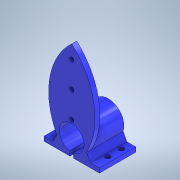
# Autodesk Inventor part: Soporte_MotorDC
Saved by Autodesk Inventor 2022 (Build 260153000, 153)
## iProperties
Created: 2022-01-28
Part Number: Soporte_MotorDC
Material: ABS Plastic
Document SubType Name: Modeling
Designer: hurta
Density: 1.06 g/cm^3
Appearance: Blue - Wall Paint - Glossy
Author: hurta
Autodesk Inventor part; units mm, degrees
ref_plane "YZ Plane" through (0, 0, 0) normal (1, 0, 0) x (0, 1, 0)
ref_plane "XZ Plane" through (0, 0, 0) normal (0, 1, 0) x (-1, 0, 0)
ref_plane "XY Plane" through (0, 0, 0) normal (0, 0, 1) x (1, 0, 0)
sketch "Sketch1" plane through (0, 0, 0) normal (0, 0, 1) x (1, 0, 0)
  line L0 (10.7443, -13.75) -> (30.7443, -13.75)
  line L1 (30.7443, -13.75) -> (30.7443, -18.75)
  line L2 (-30.7443, -13.75) -> (-10.7443, -13.75)
  circle A0 centre (0, 0) radius 13.75
  arc A1 (10.7443, -13.75) -> (-10.7443, -13.75) centre (0, 0) ccw
  line L3 (-10.7443, -13.75) -> (10.7443, -13.75) construction
  line L4 (30.7443, -18.75) -> (-30.7443, -18.75)
  line L5 (-30.7443, -18.75) -> (-30.7443, -13.75)
  point P0 (-13.75, 0)
  dimension "d6" = 27.5
  dimension "d1" = 5
  dimension "d4" = 34.9
  dimension "d7" = 20
  constraints: 12 end point, 5 horizontal, 3 horizontal alignment, 2 coincident, 2 perpendicular, 2 point on circle, 1 centre point, 1 collinear, 2 other
  measures "d1" distance of L0.end L1.end
  measures "d4" diameter of A1
  measures "d7" distance of L2.start L2.end
extrude "Extrusion1" add sketch "Sketch1" along normal blind 35
sketch "Sketch2" plane through (-30.7443, -18.75, 0) normal (0, -1, 0) x (1, 0, 0)
  line L0 (0, 35) -> (61.4886, 35) projected
  line L1 (0, 0) -> (61.4886, 0) projected
  point P0 (30.7443, 0)
  point P1 (6.1489, 25)
  point P2 (55.3397, 25)
  point P3 (6.1489, 10)
  point P4 (55.3397, 10)
  dimension "d10" = 24.5954
  dimension "d11" = 61.4886
  dimension "d12" = 24.5954
  dimension "d13" = 10
  dimension "d14" = 10
  constraints: 2 horizontal alignment, 2 vertical alignment
  measures "d10" horizontal distance of point (6.149, 25) point (30.744, 0)
  measures "d11" distance of L0.start L0.end
  measures "d12" horizontal distance of point (30.744, 0) point (55.34, 25)
  measures "d13" distance from line of L0 point (6.149, 25)
  measures "d14" distance from line of L1 point (55.34, 10)
hole "Hole1" at (-24.5954, -18.75, 25) at (24.5954, -18.75, 25) at (-24.5954, -18.75, 10) at (24.5954, -18.75, 10) direction (0, 1, 0) diameter 5.5 end through all clearance for "Flat Head Machine Screw" size "M5" standard "Ansi Metric M Profile"
sketch "Sketch3" plane through (0, 0, 35) normal (0, 0, 1) x (1, 0, 0)
  line L0 (-2, -11.7546) -> (2, -11.7546)
  line L1 (2, -11.7546) -> (2, -18.75)
  line L2 (2, -18.75) -> (-2, -18.75)
  line L3 (-2, -18.75) -> (-2, -11.7546)
  line L4 (-30.7443, -18.75) -> (30.7443, -18.75) projected
  point P0 (0, 0)
  dimension "d22" = 2
  dimension "d23" = 2
  constraints: 8 end point, 2 parallel, 1 collinear, 1 horizontal, 1 perpendicular
  measures "d22" distance from line of point (0, 0) L1
  measures "d23" distance from line of point (0, 0) L3
extrude "Extrusion2" cut sketch "Sketch3" against normal through all
chamfer "Chamfer1" distance 10 angle 45 1 edges at (10.7443, -13.75, 17.5)
chamfer "Chamfer2" distance 10 angle 45 1 edges at (-10.7443, -13.75, 17.5)
sketch "Sketch4" plane through (0, 0, 35) normal (0, 0, 1) x (1, 0, 0)
  circle A0 centre (0, 17.45) radius 2.4
  circle A1 centre (0, 46.45) radius 2.4
  line L0 (2, -18.75) -> (30.7443, -18.75) projected
  arc A2 (16.5293, -5.5932) -> (-16.5293, -5.5932) centre (0, 0) ccw projected
  arc A3 (0, 90.45) -> (-16.5293, -5.5932) centre (54.2638, 31.6671) ccw
  arc A4 (16.5293, -5.5932) -> (0, 90.45) centre (-54.2638, 31.6671) ccw
  arc A5 (16.5293, -5.5932) -> (-16.5293, -5.5932) centre (0, 0) ccw projected
  arc A6 (2, -13.6038) -> (-2, -13.6038) centre (0, 0) ccw projected
  line L1 (-2, -18.75) -> (-2, -13.6038) projected
  line L2 (2, -13.6038) -> (2, -18.75) projected
  line L3 (30.7443, -18.75) -> (30.7443, -13.75) projected
  line L4 (30.7443, -13.75) -> (20.7443, -13.75) projected
  line L5 (16.5293, -5.5932) -> (20.7443, -13.75) projected
  line L6 (-20.7443, -13.75) -> (-16.5293, -5.5932) projected
  line L7 (-20.7443, -13.75) -> (-30.7443, -13.75) projected
  line L8 (-30.7443, -13.75) -> (-30.7443, -18.75) projected
  line L9 (-30.7443, -18.75) -> (-2, -18.75) projected
  circle A7 centre (0, 75.45) radius 2.4
  point P0 (16.5293, -5.5932)
  point P1 (-16.5293, -5.5932)
  dimension "d32" = 4.8
  dimension "d33" = 4.8
  dimension "d34" = 36.2
  dimension "d35" = 29
  dimension "d38" = 80
  dimension "d51" = 4.8
  dimension "d52" = 29
  dimension "d53" = 15
  dimension "d54" = 80
  constraints: 7 point on circle, 5 centre point, 4 vertical alignment, 3 coincident
  measures "d32" diameter of A0
  measures "d33" diameter of A1
  measures "d34" distance from line of L0 A0.centre
  measures "d35" distance of A1.centre A0.centre
  measures "d38" radius of A4
  measures "d51" diameter of A7
  measures "d52" distance of A1.centre A7.centre
  measures "d53" distance of A3.start A7.centre
  measures "d54" radius of A3
extrude "Extrusion3" add sketch "Sketch4" along normal blind 5.5 contours A0 A2 A3 A4 | A0 A2 L5 L4 L3 L0 L2 A6 L1 L9 L8 L7 L6
sketch "Sketch5" plane through (0, 0, 40.5) normal (0, 0, 1) x (1, 0, 0)
  circle A0 centre (0, 17.45) radius 2.4 projected
  circle A1 centre (0, 17.45) radius 3.75
  line L0 (-2.8814, 15.05) -> (2.8814, 15.05)
  point P0 (0, 0)
  point P1 (0, 15.05)
  point P2 (-1.8933, 15.975)
  dimension "d41" = 7.5
  constraints: 2 end point, 2 point on circle, 1 centre point, 1 coincident, 1 horizontal, 1 tangent
  measures "d41" diameter of A1
extrude "Extrusion4" add sketch "Sketch5" against normal blind 25 contours L0 A1 picked at (3.2642, 17.7468)
sketch "Sketch6" plane through (0, 0, 40.5) normal (0, 0, 1) x (1, 0, 0)
  circle A0 centre (0, 17.45) radius 2.4 projected
  point P0 (0, 0)
  constraints: 1 coincident
hole "Hole2" at (0, 17.45, 40.5) direction (0, 0, -1) diameter 4.8 depth 25 tip angle 118
equation "\"d4\" = d3 + 0.5 * d0"
equation "\"d10\" = 0.4 * d11"
equation "\"d12\" = d10"
equation "\"d14\" = d13"
equation "\"d23\" = d22"
equation "\"d38\" = d54"
equation "\"d52\" = d35"
equation "\"d3\" = 27.4"
equation "\"d0\" = 15"
body "Solid1"
